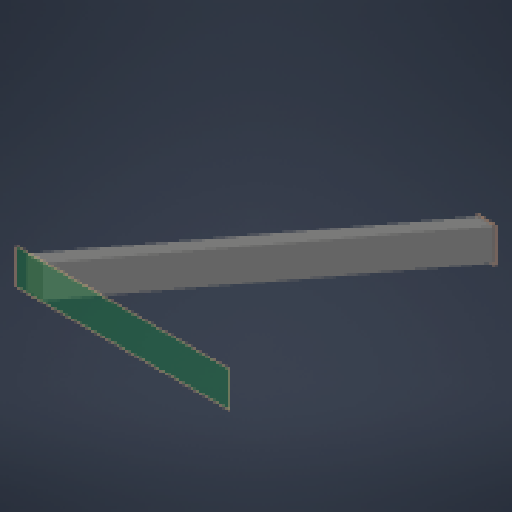
# Autodesk Inventor part: LowerEarDiagonals
Saved by Autodesk Inventor 2027 (Build 310192000, 192)
## iProperties
Created: 2026-08-07
Part Number: LowerEarDiagonals
Material: Generic
Document SubType Name: Modeling
Designer: lucas
Density: 1 g/cm^3
Appearance: Default
Author: lucas
Autodesk Inventor part; units mm, degrees
ref_plane "YZ Plane" through (0, 0, 0) normal (1, 0, 0) x (0, 1, 0)
ref_plane "XZ Plane" through (0, 0, 0) normal (0, 1, 0) x (-1, 0, 0)
ref_plane "XY Plane" through (0, 0, 0) normal (0, 0, 1) x (1, 0, 0)
ref_plane "Work Plane1" through (0, 0, 0) normal (0, 0, 1) x (1, 0, 0)
sketch "Sketch1" plane through (0, 0, 0) normal (0, 0, 1) x (1, 0, 0)
  line L0 (0, 0) -> (0, 101.6) projected
  line L1 (0, 101.6) -> (-50.8, 101.6) projected
  line L2 (-50.8, 0) -> (-50.8, 101.6) projected
  line L3 (0, 0) -> (-50.8, 0) projected
  line L4 (0, 101.6) -> (-50.8, 101.6)
  line L5 (-50.8, 101.6) -> (-50.8, 0)
  line L6 (-50.8, 0) -> (0, 0)
  line L7 (0, 0) -> (0, 101.6)
  constraints: 8 end point, 2 parallel, 1 horizontal, 1 perpendicular
ref_plane "Work Plane2" through (-355.6, 50.8, 812.8) normal (0, 0, -1) x (-1, 0, 0)
sketch "Sketch2" plane through (-355.6, 50.8, 812.8) normal (0, 0, -1) x (-1, 0, 0)
  line L0 (-304.8, -50.8) -> (304.8, -50.8) projected
  line L1 (304.8, -50.8) -> (254, -50.8)
  line L2 (254, -50.8) -> (254, 50.8)
  line L3 (254, 50.8) -> (304.8, 50.8)
  line L4 (304.8, 50.8) -> (304.8, -50.8)
  point P0 (-355.6, -50.8)
  dimension "d0" = 101.6
  dimension "d1" = 50.8
  constraints: 8 end point, 2 parallel, 1 horizontal, 1 perpendicular
  measures "d0" distance of L1.end L2.end
  measures "d1" distance of L2.end L3.end
loft "Loft1" add profiles "Sketch2", "Sketch1"
body "Solid1"
